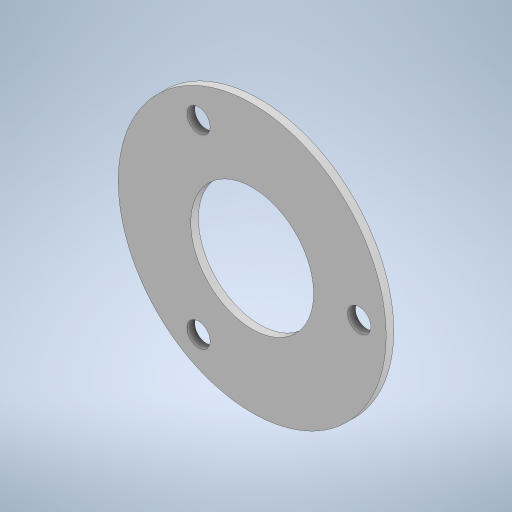
# Autodesk Inventor part: платик крепежный
Saved by Autodesk Inventor 2024.2 (Build 282272000, 272)
## iProperties
Created: 2024-04-17
Part Number: платик крепежный
Material: Generic
Document SubType Name: Sheet Metal
Designer: admin
Density: 1 g/cm^3
Sheet Metal Rule: Default
Appearance: Default
Flat Pattern Width: 7 cm
Flat Pattern Length: 7 cm
Flat Pattern Area: 49 cm^2
Sheet Metal Width: 70,000 mm
Sheet Metal Length: 70,000 mm
Sheet Metal Area: 4900,000 mm^2
Author: admin
Autodesk Inventor part; units mm, degrees
ref_plane "YZ Plane" through (0, 0, 0) normal (1, 0, 0) x (0, 1, 0)
ref_plane "XZ Plane" through (0, 0, 0) normal (0, 1, 0) x (-1, 0, 0)
ref_plane "XY Plane" through (0, 0, 0) normal (0, 0, 1) x (1, 0, 0)
sketch "Sketch1" plane through (0, 0, 0) normal (0, 0, 1) x (1, 0, 0)
  circle A0 centre (0, 0) radius 35
  dimension "d0" = 70
  measures "d0" diameter of A0
extrude "Plate1" add sketch "Sketch1" along normal blind 2
sketch "Sketch2" plane through (0, 0, 0) normal (0, 0, 1) x (1, 0, 0)
  point P0 (0, 0)
  point P1 (28, 0)
  dimension "d2" = 28
  constraints: 1 horizontal alignment
  measures "d2" distance of point (0, 0) point (28, 0)
hole "Hole1" at (28, 0, 0) direction (0, 0, 1) diameter 6 end through all
pattern_circular "Circular Pattern1" count 3 over 360 about axis through (0, 0, -10) along (0, 0, 1) of "Hole1"
sketch "Sketch3" plane through (0, 0, 2) normal (0, 0, 1) x (1, 0, 0)
  circle A0 centre (0, 0) radius 16.05
  dimension "d13" = 32.1
  constraints: 1 centre point, 1 coincident
  measures "d13" diameter of A0
extrude "Extrusion1" cut sketch "Sketch3" against normal through all
equation "\"d0\" = Внешний_диам_фланца"
equation "\"d8\" = Thickness"
equation "\"d1\" = Thickness"
equation "\"BendRadius\" = Thickness"
equation "\"BendReliefWidth\" = Thickness"
equation "\"BendReliefDepth\" = 0.5 * Thickness"
equation "\"CornerReliefSize\" = 4 * Thickness"
equation "\"MinimumRemnant\" = 2 * Thickness"
equation "\"TransitionRadius\" = BendRadius"
equation "\"JacobiRadiusSize\" = BendRadius"
equation "\"GapSize\" = Thickness"
equation "\"Внешний_диам_фланца\" = 70"
equation "\"Thickness\" = 2"
body "Solid1"
